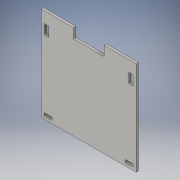
# Autodesk Inventor part: RTS Frame Front Panel
Saved by Autodesk Inventor 2016 (Build 200138000, 138)
## iProperties
Created: 2017-11-15
Part Number: RTS Frame Front Panel
Material: Generic
Document SubType Name: Modeling
Designer: student
Density: 1 g/cm^3
Appearance: Default
Author: student
Autodesk Inventor part; units mm, degrees
ref_plane "YZ Plane" through (0, 0, 0) normal (1, 0, 0) x (0, 1, 0)
ref_plane "XZ Plane" through (0, 0, 0) normal (0, 1, 0) x (-1, 0, 0)
ref_plane "XY Plane" through (0, 0, 0) normal (0, 0, 1) x (1, 0, 0)
sketch "Sketch1" plane through (0, 0, 0) normal (0, 0, 1) x (1, 0, 0)
  line L0 (49.8602, 49.276) -> (49.8602, -49.276)
  line L1 (49.8602, -49.276) -> (-49.7078, -49.276)
  line L2 (-49.7078, -49.276) -> (-49.7078, 49.276)
  line L3 (49.8602, 49.276) -> (16.0782, 49.276)
  line L4 (16.0782, 49.276) -> (16.0782, 39.116)
  line L5 (16.0782, 39.116) -> (-15.9258, 39.116)
  line L6 (-15.9258, 39.116) -> (-15.9258, 49.276)
  line L7 (-49.7078, 49.276) -> (-15.9258, 49.276)
  line L8 (16.0782, 49.276) -> (49.8602, 49.276)
  line L9 (-46.5164, 37.846) -> (-41.7666, 37.846)
  line L10 (-41.7666, 37.846) -> (-41.7666, 27.813)
  line L11 (-41.7666, 27.813) -> (-46.5164, 27.813)
  line L12 (-46.5164, 27.813) -> (-46.5164, 37.846)
  line L13 (42.037, 37.846) -> (46.7868, 37.846)
  line L14 (46.7868, 37.846) -> (46.7868, 27.813)
  line L15 (46.7868, 27.813) -> (42.037, 27.813)
  line L16 (42.037, 27.813) -> (42.037, 37.846)
  line L17 (-46.5926, -43.2793) -> (-46.5926, -46.0733)
  line L18 (-46.5926, -43.2793) -> (-38.4646, -43.2793)
  line L19 (-38.4646, -43.2793) -> (-38.4646, -46.0733)
  line L20 (-38.4646, -46.0733) -> (-46.5926, -46.0733)
  line L21 (46.5926, -43.2793) -> (38.4646, -43.2793)
  line L22 (38.4646, -43.2793) -> (38.4646, -46.0733)
  line L23 (38.4646, -46.0733) -> (46.5926, -46.0733)
  line L24 (46.5926, -43.2793) -> (46.5926, -46.0733)
  point P0 (0, 0)
  dimension "d0" = 99.568
  dimension "d1" = 98.552
  dimension "d2" = 33.782
  dimension "d3" = 10.16
  dimension "d4" = 32.004
  dimension "d9" = 4.7498
  dimension "d10" = 10.033
  dimension "d12" = 3.1914
  dimension "d13" = 4.7498
  dimension "d14" = 10.033
  dimension "d23" = 8.128
  dimension "d25" = 2.794
  constraints: 50 end point, 10 perpendicular, 7 parallel, 5 horizontal, 1 vertical
  measures "d0" distance of L0.end L1.end
  measures "d1" distance of L0.start L0.end
  measures "d2" distance of L0.start L3.end
  measures "d3" distance of L3.end L4.end
  measures "d4" distance of L4.end L5.end
  measures "d9" distance of L10.end L11.end
  measures "d10" distance of L9.end L10.end
  measures "d12" distance between parallel lines of L2 L12
  measures "d13" distance of L14.end L15.end
  measures "d14" distance of L14.start L14.end
  measures "d23" distance of L17.start L18.end
  measures "d25" distance of L18.end L19.end
extrude "Extrusion3" add sketch "Sketch1" along normal blind 2.54
body "Solid3"
